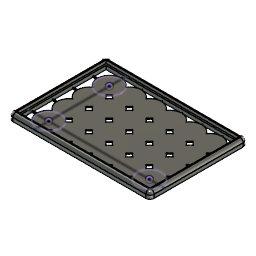
Darkfield 24 3.0 (Autodesk Fusion 360 design; units mm, degrees)
Autodesk Fusion 360 part; units mm, degrees
sketch "Sketch1" plane through (0, 0, 0) normal (0, 0, 1) x (1, 0, 0)
  line L0 (0, 0) -> (127.6, 0)
  line L1 (127.6, 0) -> (127.6, 85.5)
  line L2 (127.6, 85.5) -> (0, 85.5)
  line L3 (0, 85.5) -> (0, 0)
  dimension "d1" = 127.6
  dimension "d2" = 85.5
  constraint horizontal L0
  constraint vertical L1
  constraint horizontal L2
  constraint vertical L3
  constraint coincident L0.start L3.end
  measures "d1" distance of L0.start L0.end
  measures "d2" distance of L0.start L2.end
ref_plane "WorkPlane1" through (0, 0, 0) normal (0, -1, 0) x (1, 0, 0)
sketch "Sketch2" plane through (0, 0, 0) normal (0, -1, 0) x (1, 0, 0)
  line L0 (0, 0) -> (0, 3)
  line L1 (0, 3) -> (-3.9, 3)
  line L2 (-3.9, 3) -> (-3.9, -3.5)
  line L3 (-3.9, -3.5) -> (1.6, -3.5)
  line L4 (1.6, -3.5) -> (1.6, 0)
  line L5 (0, 0) -> (1.6, 0)
  line L6 (-3.9, -2.5) -> (1.6, -2.5)
  line L7 (0, 0) -> (127.6, 0)
  dimension "d4" = 3
  dimension "d6" = 1
  dimension "d7" = 2.5
  dimension "d8" = 3.9
  dimension "d9" = 5.5
  constraint coincident L0.start L5.start
  constraint vertical L0
  constraint perpendicular L0 L1
  constraint perpendicular L1 L2
  constraint perpendicular L2 L3
  constraint perpendicular L1 L4
  constraint perpendicular L4 L5
  constraint coincident L2 L6.start
  constraint coincident L4 L6.end
  constraint perpendicular L4 L6
  measures "d4" distance of L0.start L0.end
  measures "d6" distance of L3 L6
  measures "d7" distance of L6 L7
  measures "d8" distance of L0 L2
  measures "d9" distance of L2 L4
sweep "Sweep1" add profiles "Sketch2" path "Sketch1" along L3 L0 L1 L2 section 1 makes body 1
sketch "Sketch3" plane through (0, 0, -3.5) normal (0, 0, 1) x (-1, 0, 0)
  line L0 (0, 0) -> (-127.6, 0)
  line L1 (-127.6, 0) -> (-127.6, -85.5)
  line L2 (-127.6, -85.5) -> (0, -85.5)
  line L3 (0, -85.5) -> (0, 0)
  line L4 (-126, -1.6) -> (-1.6, -1.6)
  line L5 (-1.6, -1.6) -> (-1.6, -83.9)
  line L6 (-1.6, -83.9) -> (-126, -83.9)
  line L7 (-126, -83.9) -> (-126, -1.6)
  circle A0 centre (-17, -13.6) radius 11.5
  line L8 (3.9, 3.9) -> (3.9, -89.4)
  line L9 (3.9, -89.4) -> (-131.5, -89.4)
  line L10 (-131.5, -89.4) -> (-131.5, 3.9)
  line L11 (-131.5, 3.9) -> (3.9, 3.9)
  line L12 (-126, -1.6) -> (-126, -83.9)
  line L13 (-126, -83.9) -> (-1.6, -83.9)
  line L14 (-1.6, -83.9) -> (-1.6, -1.6)
  line L15 (-1.6, -1.6) -> (-126, -1.6)
  dimension "d16" = 17
  dimension "d17" = 13.6
  dimension "d18" = 23
  measures "d16" distance of L3 A0.centre
  measures "d17" distance of L0 A0.centre
  measures "d18" diameter of A0
extrude "Extrude1" add sketch "Sketch3" along normal blind 1 separate body contours A0 makes body 2
pattern_linear "R-Pattern1" count 6 spacing 19.28 along (1, 0, 0) count 4 spacing 19.3333 along (0, 1, 0) of bodies 2 makes body 3 at (33.89, 16.597, -3.5) makes body 4 at (53.17, 16.597, -3.5) makes body 5 at (72.45, 16.597, -3.5) makes body 6 at (91.73, 16.597, -3.5) makes body 7 at (111.01, 16.597, -3.5) makes body 8 at (13.1277, 34.5966, -3.5) makes body 9 at (32.9538, 32.9713, -3.5) makes body 10 at (52.2338, 32.9713, -3.5) makes body 11 at (71.5138, 32.9713, -3.5) makes body 12 at (90.7938, 32.9713, -3.5) makes body 13 at (110.0738, 32.9713, -3.5) makes body 14 at (18.8943, 50.2991, -3.5) makes body 15 at (33.8471, 49.841, -3.5) makes body 16 at (53.1271, 49.841, -3.5) makes body 17 at (72.4071, 49.841, -3.5) makes body 18 at (91.6871, 49.841, -3.5) makes body 19 at (110.9671, 49.841, -3.5) makes body 20 at (18.8943, 69.6325, -3.5) makes body 21 at (33.8471, 69.1743, -3.5) makes body 22 at (53.1271, 69.1743, -3.5) makes body 23 at (72.4071, 69.1743, -3.5) makes body 24 at (91.6871, 69.1743, -3.5) makes body 25 at (110.9671, 69.1743, -3.5)
sketch "Sketch4" plane through (0, 0, -2.5) normal (0, 0, 1) x (-1, 0, 0)
  circle A0 centre (-36.28, -71.6) radius 11.5
  circle A1 centre (-17, -71.6) radius 11.5
  circle A2 centre (-17, -52.2667) radius 11.5
  dimension "d64" = 19.28
  dimension "d65" = 19.3333
  measures "d64" distance of A0.centre A1.centre
  measures "d65" distance of A1.centre A2.centre
ref_plane "WorkPlane2" through (63.8, 42.75, -0.25) normal (-1, 0, 0) x (0, 0, -1)
ref_plane "WorkPlane3" through (63.8, 42.75, -0.25) normal (0, -1, 0) x (0, 0, -1)
ref_plane "WorkPlane4" through (-3.9, -3.9, -3.5) normal (0.567406, -0.823438, 0) x (0.823438, 0.567406, 0)
sketch "Sketch5" plane through (0, 0, -3.5) normal (0, 0, -1) x (1, 0, 0)
  line L0 (-3.9, 3.9) -> (-3.9, -89.4)
  line L1 (-3.9, -89.4) -> (131.5, -89.4)
  line L2 (131.5, -89.4) -> (131.5, 3.9)
  line L3 (131.5, 3.9) -> (-3.9, 3.9)
  line L4 (126, -1.6) -> (126, -83.9)
  line L5 (126, -83.9) -> (1.6, -83.9)
  line L6 (1.6, -83.9) -> (1.6, -1.6)
  line L7 (1.6, -1.6) -> (126, -1.6)
  line L8 (17, -13.1) -> (113.4, -13.1)
  line L9 (113.4, -13.1) -> (113.4, -14.1)
  line L10 (113.4, -14.1) -> (17, -14.1)
  line L11 (17, -14.1) -> (17, -13.1)
  line L12 (16.5, -13.6) -> (17.5, -13.6)
  line L13 (17.5, -13.6) -> (17.5, -71.6)
  line L14 (17.5, -71.6) -> (16.5, -71.6)
  line L15 (16.5, -71.6) -> (16.5, -13.6)
  circle A0 centre (17, -13.6) radius 11.5
  circle A1 centre (17, -71.6) radius 11.5
  circle A2 centre (113.4, -13.6) radius 11.5
  line L16 (16.5, -13.6) -> (17.5, -13.6)
  line L17 (17.5, -13.6) -> (17.5, 1.8131)
  line L18 (17.5, 1.8131) -> (16.5, 1.8131)
  line L19 (16.5, 1.8131) -> (16.5, -13.6)
  line L20 (16.5, -71.6) -> (17.5, -71.6)
  line L21 (17.5, -71.6) -> (17.5, -87)
  line L22 (17.5, -87) -> (16.5, -87)
  line L23 (16.5, -87) -> (16.5, -71.6)
  line L24 (113.4, -13.1) -> (129.0228, -13.1)
  line L25 (129.0228, -13.1) -> (129.0228, -14.1)
  line L26 (129.0228, -14.1) -> (113.4, -14.1)
  line L27 (113.4, -14.1) -> (113.4, -13.1)
  line L28 (17, -13.1) -> (-2.5, -13.1)
  line L29 (-2.5, -13.1) -> (-2.5, -14.1)
  line L30 (-2.5, -14.1) -> (17, -14.1)
  line L31 (17, -14.1) -> (17, -13.1)
  dimension "d39" = 1
  dimension "d40" = 1
  dimension "d41" = 58
  dimension "d42" = 96.4
  constraint horizontal L8
  constraint vertical L9
  constraint horizontal L10
  constraint vertical L11
  constraint midpoint L11 A0.centre
  constraint horizontal L12
  constraint vertical L13
  constraint horizontal L14
  constraint vertical L15
  constraint midpoint L14 A1.centre
  constraint midpoint L12 A0.centre
  constraint midpoint L9 A2.centre
  constraint horizontal L16
  constraint vertical L17
  constraint horizontal L18
  constraint vertical L19
  constraint coincident L12.end L13.start
  constraint horizontal L20
  constraint vertical L21
  constraint horizontal L22
  constraint vertical L23
  constraint horizontal L24
  constraint vertical L25
  constraint horizontal L26
  constraint vertical L27
  constraint coincident L9.end L10.start
  constraint coincident L13.end L14.start
  constraint horizontal L28
  constraint vertical L29
  constraint horizontal L30
  constraint vertical L31
  constraint coincident L10.end L11.start
  measures "d39" distance of L8.start L10.end
  measures "d40" distance of L12.start L12.end
  measures "d41" distance of L12.start L14.end
  measures "d42" distance of L8.start L8.end
extrude "Extrude2" add sketch "Sketch5" against normal blind 1 separate body contours L7 A0 L17 L19 | L7 L17 L18 L19 | L8 A0 L17 L19 L28 | L8 L11 L12 L16 L17 L31 | L5 L21 L22 L23 | L5 A1 L21 L23 | L11 L12 L16 L19 L28 L31 | L10 L11 L12 L13 L16 L31 | L14 A1 L20 L21 L23 | L11 L12 L15 L16 L30 L31 | L10 L13 L15 A0 L30 | L13 L14 L15 A1 L20 | L13 L15 A0 A1 makes body 26
extrude "Extrude3" add sketch "Sketch5" against normal blind 1 separate body contours L4 L24 L25 L26 | L4 A2 L24 L26 | L9 A2 L24 L26 L27 | L8 L10 A0 A2 | L8 L9 L10 A2 L27 | L8 L10 L13 A0 L17 | L8 L11 L12 L16 L17 L31 | L6 A0 L28 L30 | L6 L28 L29 L30 | L15 A0 L19 L28 L30 | L11 L12 L16 L19 L28 L31 | L10 L11 L12 L13 L16 L31 | L11 L12 L15 L16 L30 L31 makes body 27
pattern_linear "R-Pattern5" count 4 spacing 19.3333 along (0, 1, 0) of bodies 27 makes body 28 at (77.437, 33.1, -3.5) makes body 29 at (77.437, 52.4333, -3.5) makes body 30 at (77.437, 71.7667, -3.5)
pattern_linear "R-Pattern4" count 6 spacing 19.28 along (1, 0, 0) of bodies 26 makes body 31 at (36.4467, 48.437, -3.5) makes body 32 at (55.7267, 48.437, -3.5) makes body 33 at (74.6733, 36.763, -3.5) makes body 34 at (93.9533, 36.763, -3.5) makes body 35 at (113.2333, 36.763, -3.5)
combine "Combine1" operation add target body 1 tool bodies 7 35 8 21 22 11 5 34 15 28 14 29 2 30 3 27 20 4 19 18 25 33 23 17 32 16 6 12 10 24 13 26 9 31
fillet "Fillet1" radius 4 4 edges at (-3.9, -3.9, -0.25) (-3.9, 89.4, -0.25) (131.5, 89.4, -0.25) (131.5, -3.9, -0.25) on bodies 1
fillet "Fillet2" radius 3 8 edges at (130.3284, -2.7284, 3) (131.5, 42.75, 3) (130.3284, 88.2284, 3) (63.8, 89.4, 3) (-2.7284, 88.2284, 3) (-3.9, 42.75, 3) (-2.7284, -2.7284, 3) (63.8, -3.9, 3) on bodies 1
equation "d6 = mask_thickness"
equation "d7 = plate_mask_dist"
equation "d18 = mask_dia"
equation "d19 = mask_thickness"
equation "d23 = 113.4 mm - 17 mm"
equation "d24 = -13.6 mm + 71.6 mm"
equation "d47 = -d42"
equation "d53 = d41"
equation "mask_dia = 15.6 mm + 3.4 mm + 2 mm + 1 mm + 1 mm"
equation "mask_thickness = 1 mm"
equation "plate_mask_dist = 2.5 mm"
named bodies: "24WellMask"
